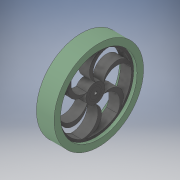
# Autodesk Inventor part: Wheel
Saved by Autodesk Inventor 2018 (Build 220112000, 112)
## iProperties
Created: 2018-10-12
Part Number: Wheel
Material: Generic
Document SubType Name: Modeling
Designer: 566609
Density: 1 g/cm^3
Appearance: Default
Author: 566609
Autodesk Inventor part; units mm, degrees
ref_plane "YZ Plane" through (0, 0, 0) normal (1, 0, 0) x (0, 1, 0)
ref_plane "XZ Plane" through (0, 0, 0) normal (0, 1, 0) x (-1, 0, 0)
ref_plane "XY Plane" through (0, 0, 0) normal (0, 0, 1) x (1, 0, 0)
sketch "Sketch1" plane through (0, 0, 0) normal (1, 0, 0) x (0, 1, 0)
  circle A0 centre (0, 0) radius 50.8
  circle A1 centre (0, 0) radius 40.8
  circle A2 centre (0, 0) radius 10.8
  circle A3 centre (0, 0) radius 5.8
  dimension "d0" = 101.6
  dimension "d1" = 10
  dimension "d2" = 30
  dimension "d3" = 5
  constraints: 4 centre point, 1 coincident
  measures "d0" diameter of A0
  measures "d1" radial gap between concentric circles of A0 A1
  measures "d2" radial gap between concentric circles of A1 A2
  measures "d3" radial gap between concentric circles of A2 A3
extrude "Extrusion1" add sketch "Sketch1" along normal mid plane 20
sketch "Sketch2" plane through (10, 0, 0) normal (1, 0, 0) x (0, 0, -1)
  circle A0 centre (0, 0) radius 40.8 projected
  circle A1 centre (0, 0) radius 10.8 projected
  arc A2 (15.6051, 37.6978) -> (0, 10.8) centre (8.6314, 23.768) ccw
  arc A3 (15.6051, 37.6978) -> (0, 10.8) centre (14.4186, 20.4105) ccw
  arc A4 (40.4498, 5.3344) -> (9.3531, 5.4) centre (24.8994, 4.409) ccw
  arc A5 (40.4498, 5.3344) -> (9.3531, 5.4) centre (24.8853, -2.2817) ccw
  arc A6 (24.8447, -32.3633) -> (9.3531, -5.4) centre (16.268, -19.359) ccw
  arc A7 (24.8447, -32.3633) -> (9.3531, -5.4) centre (10.4667, -22.6921) ccw
  arc A8 (-15.6051, -37.6978) -> (0, -10.8) centre (-8.6314, -23.768) ccw
  arc A9 (-15.6051, -37.6978) -> (0, -10.8) centre (-14.4186, -20.4105) ccw
  arc A10 (-40.4498, -5.3344) -> (-9.3531, -5.4) centre (-24.8994, -4.409) ccw
  arc A11 (-40.4498, -5.3344) -> (-9.3531, -5.4) centre (-24.8853, 2.2817) ccw
  arc A12 (-24.8447, 32.3633) -> (-9.3531, 5.4) centre (-16.268, 19.359) ccw
  arc A13 (-24.8447, 32.3633) -> (-9.3531, 5.4) centre (-10.4667, 22.6921) ccw
  dimension "d8" = 360
  constraints: 24 point on circle, 12 centre point, 1 vertical alignment, 40 other
extrude "Extrusion2" add sketch "Sketch2" against normal blind 20 contours A5 A4 A0 | A0 A4 | A6 A0 | A0 A7 A6 | A3 A2 A0 | A0 A2 | A8 A0 | A0 A9 A8 | A12 A0 A13 | A10 A0 A11 | A0 A12 | A10 A0
sketch "Sketch3" plane through (10, 0, 0) normal (1, 0, 0) x (0, 0, -1)
  circle A0 centre (0, 0) radius 43.4
  dimension "d12" = 86.8
  constraints: 1 centre point, 1 coincident
  measures "d12" diameter of A0
extrude "Extrusion3" cut sketch "Sketch3" against normal blind 3.81
sketch "Sketch4" plane through (-10, 0, 0) normal (-1, 0, 0) x (0, 0, 1)
  circle A0 centre (0, 0) radius 43.3959
  dimension "d15" = 86.7918
  constraints: 1 centre point, 1 coincident
  measures "d15" diameter of A0
extrude "Extrusion4" cut sketch "Sketch4" against normal blind 3.81
sketch "Sketch5" plane through (6.19, 0, 0) normal (1, 0, 0) x (0, 0, -1)
  line L0 (0.3556, 1.4986) -> (-0.3556, 1.4986)
  line L1 (-1.4986, 0.3556) -> (-1.4986, -0.3556)
  line L2 (-0.3556, -1.4986) -> (0.3556, -1.4986)
  line L3 (1.4986, -0.3556) -> (1.4986, 0.3556)
  arc A0 (-0.3556, 1.4986) -> (-1.4986, 0.3556) centre (-0.3556, 0.3556) ccw
  arc A1 (1.4986, 0.3556) -> (0.3556, 1.4986) centre (0.3556, 0.3556) ccw
  arc A2 (0.3556, -1.4986) -> (1.4986, -0.3556) centre (0.3556, -0.3556) ccw
  arc A3 (-1.4986, -0.3556) -> (-0.3556, -1.4986) centre (-0.3556, -0.3556) ccw
  line L4 (0.3556, 7.4499) -> (-0.3556, 7.4499)
  arc A4 (-0.3556, 7.4499) -> (-7.4499, 0.3556) centre (-0.3556, 0.3556) ccw
  line L5 (-7.4499, 0.3556) -> (-7.4499, -0.3556)
  arc A5 (-7.4499, -0.3556) -> (-0.3556, -7.4499) centre (-0.3556, -0.3556) ccw
  line L6 (-0.3556, -7.4499) -> (0.3556, -7.4499)
  arc A6 (0.3556, -7.4499) -> (7.4499, -0.3556) centre (0.3556, -0.3556) ccw
  line L7 (7.4499, -0.3556) -> (7.4499, 0.3556)
  arc A7 (7.4499, 0.3556) -> (0.3556, 7.4499) centre (0.3556, 0.3556) ccw
  point P0 (0, 0)
  point P1 (-1.4986, -1.4986)
  point P2 (-1.4986, 1.4986)
  point P3 (1.4986, -1.4986)
  dimension "d18" = 2.9972
  dimension "d19" = 2.9972
  dimension "d20" = 1.143
  constraints: 16 end point, 16 point on circle, 8 centre point, 8 tangent, 6 point on line, 4 parallel, 3 equal radius, 2 perpendicular, 1 horizontal, 7 other
  measures "d18" distance of point (1.499, -1.499) point (-1.499, -1.499)
  measures "d19" distance of point (-1.499, -1.499) point (-1.499, 1.499)
  measures "d20" radius of A0
extrude "Extrusion5" add sketch "Sketch5" against normal blind 12.7 separate body
body "Solid1"
body "Solid3"
